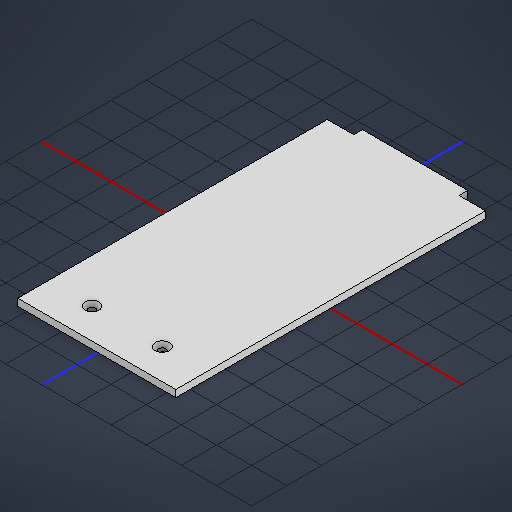
# Autodesk Inventor part: 000.005.003 - Крышка
Saved by Autodesk Inventor 2025 (Build 290162000, 162)
## iProperties
Created: 2024-08-25
Part Number: 000.005.003 - Крышка
Material: Типовые
Document SubType Name: Modeling
Designer: IvanPetrov
Density: 1 g/cm^3
Appearance: По умолчанию
Author: IvanPetrov
Autodesk Inventor part; units mm, degrees
ref_plane "YZ Plane" through (0, 0, 0) normal (1, 0, 0) x (0, 1, 0)
ref_plane "XZ Plane" through (0, 0, 0) normal (0, 1, 0) x (-1, 0, 0)
ref_plane "XY Plane" through (0, 0, 0) normal (0, 0, 1) x (1, 0, 0)
sketch "Эскиз1" plane through (0, 0, 0) normal (0, 1, 0) x (-1, 0, 0)
  line L0 (-45, 88.1475) -> (45, 88.1475)
  line L1 (45, 88.1475) -> (45, -88.1475)
  line L2 (45, -88.1475) -> (-45, -88.1475)
  line L3 (-45, -88.1475) -> (-45, 88.1475)
  line L4 (-45, 88.1475) -> (45, -88.1475) construction
  line L5 (45, 88.1475) -> (-45, -88.1475) construction
  point P0 (0, 0)
  dimension "d0" = 90
  dimension "d1" = 176.295
  constraints: 12 end point, 2 midpoint, 2 parallel, 1 horizontal, 1 perpendicular
  measures "d0" distance of L1.end L2.end
  measures "d1" distance of L0.end L1.end
extrude "Выдавливание1" add sketch "Эскиз1" along normal blind 4
sketch "Эскиз2" plane through (0, 4, 0) normal (0, 1, 0) x (1, 0, 0)
  circle A0 centre (-20, -70.8525) radius 2 projected
  circle A1 centre (20, -70.8525) radius 2 projected
  point P0 (0, 0)
extrude "Выдавливание2" cut sketch "Эскиз2" against normal through all
chamfer "Фаска1" distance 2 angle 45 2 edges at (-22, 4, 70.8525) (18, 4, 70.8525)
sketch "Эскиз3" plane through (45, 0, -88.1475) normal (0, 0, -1) x (-1, 0, 0)
  line L0 (90, 4) -> (0, 4) projected
  line L1 (90, 0) -> (0, 0) projected
  line L2 (15, 4) -> (75, 4)
  line L3 (75, 4) -> (75, 0)
  line L4 (75, 0) -> (15, 0)
  line L5 (15, 0) -> (15, 4)
  point P0 (45, 0)
  point P1 (45, 0)
  dimension "d9" = 60
  dimension "d10" = 30
  constraints: 8 end point, 2 parallel, 2 point on line, 1 horizontal, 1 midpoint, 1 perpendicular
  measures "d9" distance between parallel lines of L5 L3
  measures "d10" distance from line of point (45, 0) L5
extrude "Выдавливание3" add sketch "Эскиз3" along normal blind 5
equation "\"d10\" = 0.5 * d9"
